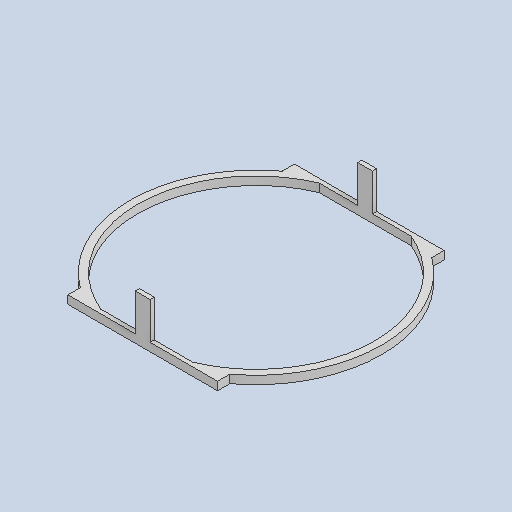
# Autodesk Inventor part: cir
Saved by Autodesk Inventor 2025 (Build 290162000, 162)
## iProperties
Created: 2025-08-16
Part Number: cir
Material: Generic
Document SubType Name: Modeling
Designer: Pravoslav
Density: 1 g/cm^3
Appearance: Default
Author: Pravoslav
Autodesk Inventor part; units mm, degrees
ref_plane "YZ Plane" through (0, 0, 0) normal (1, 0, 0) x (0, 1, 0)
ref_plane "XZ Plane" through (0, 0, 0) normal (0, 1, 0) x (-1, 0, 0)
ref_plane "XY Plane" through (0, 0, 0) normal (0, 0, 1) x (1, 0, 0)
sketch "Sketch1" plane through (0, 0, 0) normal (0, 1, 0) x (-1, 0, 0)
  circle A0 centre (0, 0) radius 30.5
  circle A1 centre (0, 0) radius 28.75
  line L0 (18.166, -27.5) -> (-18.166, -27.5)
  line L1 (-18.166, -27.5) -> (-18.166, 27.5)
  line L2 (-18.166, 27.5) -> (18.166, 27.5)
  line L3 (18.166, 27.5) -> (18.166, -27.5)
  line L4 (18.166, -27.5) -> (-18.166, 27.5) construction
  line L5 (-18.166, -27.5) -> (18.166, 27.5) construction
  line L6 (26.5, -26.5) -> (-26.5, -26.5)
  line L7 (-26.5, -26.5) -> (-26.5, 26.5)
  line L8 (-26.5, 26.5) -> (26.5, 26.5)
  line L9 (26.5, 26.5) -> (26.5, -26.5)
  line L10 (26.5, -26.5) -> (-26.5, 26.5) construction
  line L11 (-26.5, -26.5) -> (26.5, 26.5) construction
  point P0 (11.1496, -26.5)
  point P1 (-11.1496, -26.5)
  point P2 (-11.1496, 26.5)
  point P3 (11.1496, 26.5)
  point P4 (18.166, -24.4999)
  point P5 (18.166, 24.4999)
  point P6 (-18.166, 24.4999)
  point P7 (-18.166, -24.4999)
  dimension "d0" = 61
  dimension "d1" = 1.75
  dimension "d4" = 36.332
  dimension "d5" = 55
  dimension "d6" = 53
  dimension "d7" = 53
  constraints: 24 end point, 4 midpoint, 4 parallel, 2 centre point, 2 coincident, 2 horizontal, 2 perpendicular
  measures "d0" diameter of A0
  measures "d1" radial gap between concentric circles of A0 A1
  measures "d4" distance of L1.end L2.end
  measures "d5" distance of L0.end L1.end
  measures "d6" distance of L7.end L8.end
  measures "d7" distance of L6.end L7.end
extrude "Extrusion1" add sketch "Sketch1" along normal blind 2 contours A0 L9 A1 | L9 A1 L3 A0 | A0 L3 A1 L9 | L3 A1 L8 A0 | A0 L8 L3 | L3 L6 A0 | A0 L6 A1 L3 | L8 A1 L2 A0 | A0 L2 L3 L8 | L6 L3 L0 A0 | A0 L0 A1 L6 | L8 A1 L2 | A1 L0 L6 | L2 A1 L8 A0 | A0 L8 L1 L2 | A1 L1 A0 L8 | L0 L1 L6 A0 | A0 L6 A1 L0 | L6 A0 L1 A1 | A0 L1 L8 | A1 L7 A0 L1 | L6 L1 A0 | L1 A0 L7 A1 | A1 L7 A0
sketch "Sketch2" plane through (0, 2, 0) normal (0, 1, 0) x (1, 0, 0)
  line L0 (-18.166, -27.5) -> (18.166, -27.5) projected
  line L1 (11.1496, -26.5) -> (-11.1496, -26.5) projected
  line L2 (1.8, -27.5) -> (-1.8, -27.5)
  line L3 (-1.8, -27.5) -> (-1.8, -26.5)
  line L4 (-1.8, -26.5) -> (1.8, -26.5)
  line L5 (1.8, -26.5) -> (1.8, -27.5)
  point P0 (0, 0)
  point P1 (0, -26.5)
  point P2 (1.8, -27)
  dimension "d8" = 3.6
  dimension "d9" = 1.8
  constraints: 8 end point, 2 midpoint, 2 parallel, 2 point on line, 1 horizontal, 1 perpendicular
  measures "d8" distance of L3.end L4.end
  measures "d9" horizontal distance of point (0, -26.5) point (1.8, -27)
extrude "Extrusion2" add sketch "Sketch2" along normal blind 9
mirror "Mirror1" about plane through (0, 0, 0) normal (0, 0, 1) of "Extrusion2"
body "Solid1"
